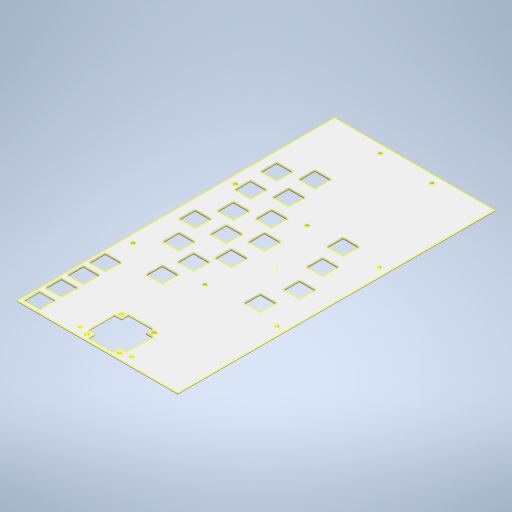
# Autodesk Inventor part: frame
Saved by Autodesk Inventor 2024 (Build 280153000, 153)
## iProperties
Created: 2023-10-17
Part Number: frame
Material: ABS 塑料
Document SubType Name: Modeling
Designer: Administrator
Density: 1.06 g/cm^3
Appearance: 白色
Author: Administrator
Autodesk Inventor part; units mm, degrees
(part 1 of 2)
ref_plane "YZ Plane" through (0, 0, 0) normal (1, 0, 0) x (0, 1, 0)
ref_plane "XY Plane" through (0, 0, 0) normal (0, 0, 1) x (1, 0, 0)
ref_plane "底层" through (0, -2, 0) normal (0, 1, 0) x (-1, 0, 0)
ref_plane "第二层" through (0, 4, 0) normal (0, 1, 0) x (-1, 0, 0)
ref_plane "第三层" through (0, 8, 0) normal (0, 1, 0) x (-1, 0, 0)
ref_plane "第四层" through (0, 12, 0) normal (0, 1, 0) x (-1, 0, 0)
sketch "第一层草图" plane through (0, 0, 0) normal (0, 1, 0) x (-1, 0, 0)
  line L0 (90, 150) -> (-90, 150)
  line L1 (-100, 140) -> (-100, -140)
  line L2 (-90, -150) -> (90, -150)
  line L3 (100, -140) -> (100, 140)
  line L4 (100, 150) -> (-100, -150) construction
  line L5 (-100, 150) -> (100, -150) construction
  arc A0 (100, 140) -> (90, 150) centre (90, 140) ccw
  arc A1 (-90, 150) -> (-100, 140) centre (-90, 140) ccw
  arc A2 (-100, -140) -> (-90, -150) centre (-90, -140) ccw
  arc A3 (90, -150) -> (100, -140) centre (90, -140) ccw
  point P0 (0, 0)
  dimension "d2" = 200
  dimension "d3" = 300
  dimension "d4" = 10
  constraints: 12 end point, 8 point on circle, 8 point on line, 8 tangent, 4 centre point, 3 equal radius, 2 midpoint, 2 parallel, 1 horizontal, 1 perpendicular
  measures "d2" distance of L5.end L4.end
  measures "d3" distance of L4.end L5.start
  measures "d4" radius of A0
sketch "第二层草图" plane through (0, 4, 0) normal (0, 1, 0) x (-1, 0, 0)
  line L0 (100, -140) -> (100, 140) projected
  line L1 (100, 0) -> (-88, 0)
  line L2 (90, 150) -> (-78, 150)
  line L3 (-88, 140) -> (-88, -140)
  line L4 (-78, -150) -> (90, -150)
  line L5 (100, -140) -> (100, 140)
  line L6 (100, 150) -> (-88, -150) construction
  line L7 (-88, 150) -> (100, -150) construction
  arc A0 (100, 140) -> (90, 150) centre (90, 140) ccw
  arc A1 (-78, 150) -> (-88, 140) centre (-78, 140) ccw
  arc A2 (-88, -140) -> (-78, -150) centre (-78, -140) ccw
  arc A3 (90, -150) -> (100, -140) centre (90, -140) ccw
  point P0 (0, 0)
  point P1 (6, 0)
  dimension "d101" = 188
  dimension "d102" = 188
  dimension "d103" = 300
  dimension "d104" = 10
  dimension "d125" = 10
  constraints: 14 end point, 8 point on circle, 8 point on line, 8 tangent, 4 centre point, 4 midpoint, 2 equal radius, 2 horizontal, 2 parallel, 1 perpendicular
  measures "d101" distance of L1.start L1.end
  measures "d102" distance of L7.end L6.end
  measures "d103" distance of L6.end L7.start
  measures "d104" radius of A0
  measures "d125" radius of A3
sketch "第三层草图" plane through (0, 8, 0) normal (0, 1, 0) x (-1, 0, 0)
  line L0 (100, -140) -> (100, 140) projected
  line L1 (100, 0) -> (-76, 0)
  line L2 (90, 150) -> (-66, 150)
  line L3 (-76, 140) -> (-76, -140)
  line L4 (-66, -150) -> (90, -150)
  line L5 (100, -140) -> (100, 140)
  line L6 (100, 150) -> (-76, -150) construction
  line L7 (-76, 150) -> (100, -150) construction
  arc A0 (100, 140) -> (90, 150) centre (90, 140) ccw
  arc A1 (-66, 150) -> (-76, 140) centre (-66, 140) ccw
  arc A2 (-76, -140) -> (-66, -150) centre (-66, -140) ccw
  arc A3 (90, -150) -> (100, -140) centre (90, -140) ccw
  point P0 (0, 0)
  point P1 (12, 0)
  dimension "d105" = 176
  dimension "d106" = 176
  dimension "d107" = 300
  dimension "d108" = 10
  constraints: 14 end point, 8 point on circle, 8 point on line, 8 tangent, 4 centre point, 4 midpoint, 3 equal radius, 2 horizontal, 2 parallel, 1 perpendicular
  measures "d105" distance of L1.start L1.end
  measures "d106" distance of L7.end L6.end
  measures "d107" distance of L6.end L7.start
  measures "d108" radius of A0
sketch "第四层草图" plane through (0, 12, 0) normal (0, 1, 0) x (-1, 0, 0)
  line L0 (100, -140) -> (100, 140) projected
  line L1 (100, 0) -> (-64, 0)
  line L2 (90, 150) -> (-54, 150)
  line L3 (-64, 140) -> (-64, -140)
  line L4 (-54, -150) -> (90, -150)
  line L5 (100, -140) -> (100, 140)
  line L6 (100, 150) -> (-64, -150) construction
  line L7 (-64, 150) -> (100, -150) construction
  arc A0 (100, 140) -> (90, 150) centre (90, 140) ccw
  arc A1 (-54, 150) -> (-64, 140) centre (-54, 140) ccw
  arc A2 (-64, -140) -> (-54, -150) centre (-54, -140) ccw
  arc A3 (90, -150) -> (100, -140) centre (90, -140) ccw
  point P0 (0, 0)
  point P1 (18, 0)
  dimension "d109" = 164
  dimension "d110" = 164
  dimension "d111" = 300
  dimension "d112" = 10
  dimension "d113" = 10
  constraints: 14 end point, 8 point on circle, 8 point on line, 8 tangent, 4 centre point, 4 midpoint, 2 equal radius, 2 horizontal, 2 parallel, 1 perpendicular
  measures "d109" distance of L1.start L1.end
  measures "d110" distance of L7.end L6.end
  measures "d111" distance of L6.end L7.start
  measures "d112" radius of A0
  measures "d113" radius of A2
sketch "底层草图" plane through (0, -2, 0) normal (0, 1, 0) x (-1, 0, 0)
  line L0 (98, 140) -> (98, -140)
  arc A0 (90, -148) -> (98, -140) centre (90, -140) ccw
  line L1 (90, -148) -> (-90, -148)
  arc A1 (-98, -140) -> (-90, -148) centre (-90, -140) ccw
  line L2 (-98, -140) -> (-98, 140)
  arc A2 (-90, 148) -> (-98, 140) centre (-90, 140) ccw
  line L3 (-90, 148) -> (90, 148)
  arc A3 (98, 140) -> (90, 148) centre (90, 140) ccw
  point P0 (0, 0)
  constraints: 8 end point, 8 point on circle, 4 centre point
extrude "拉伸25" add sketch "底层草图" along normal blind 2
extrude "拉伸26" add sketch "第一层草图" along normal blind 4 separate body
extrude "拉伸27" add sketch "第二层草图" along normal blind 4 separate body
extrude "拉伸28" add sketch "第三层草图" along normal blind 4 separate body
extrude "拉伸29" add sketch "第四层草图" along normal blind 4 separate body
sketch "草图20" plane through (0, 16, 0) normal (0, 1, 0) x (1, 0, 0)
  line L0 (-100, 140) -> (-100, -140) projected
  arc A0 (-100, -140) -> (-90, -150) centre (-90, -140) ccw projected
  line L1 (-90, -150) -> (54, -150) projected
  arc A1 (54, -150) -> (64, -140) centre (54, -140) ccw projected
  line L2 (64, -140) -> (64, 140) projected
  arc A2 (64, 140) -> (54, 150) centre (54, 140) ccw projected
  line L3 (54, 150) -> (-90, 150) projected
  arc A3 (-90, 150) -> (-100, 140) centre (-90, 140) ccw projected
  line L4 (-90, -140) -> (-92.1213, -142.1213)
  line L5 (-90, -140) -> (-87, -140) construction
  circle A4 centre (-92.1213, -142.1213) radius 2.75
  line L6 (-90, 140) -> (-92.1213, 142.1213)
  circle A5 centre (-92.1213, 142.1213) radius 2.75
  line L7 (54, -140) -> (56.1213, -142.1213)
  line L8 (54, -140) -> (57, -140) construction
  circle A6 centre (56.1213, -142.1213) radius 2.75
  line L9 (54, 140) -> (56.1213, 142.1213)
  circle A7 centre (56.1213, 142.1213) radius 2.75
  line L10 (-88, -138) -> (-88, 138)
  line L11 (-88, 138) -> (52, 138)
  line L12 (52, 138) -> (52, -138)
  line L13 (52, -138) -> (-88, -138)
  line L14 (-89.3713, -142.1213) -> (-90.7463, -144.5029)
  line L15 (-90.7463, -144.5029) -> (-93.4963, -144.5029)
  line L16 (-93.4963, -144.5029) -> (-94.8713, -142.1213)
  line L17 (-94.8713, -142.1213) -> (-93.4963, -139.7398)
  line L18 (-93.4963, -139.7398) -> (-90.7463, -139.7398)
  line L19 (-90.7463, -139.7398) -> (-89.3713, -142.1213)
  line L20 (-89.3713, 142.1213) -> (-90.7463, 139.7398)
  line L21 (-90.7463, 139.7398) -> (-93.4963, 139.7398)
  line L22 (-93.4963, 139.7398) -> (-94.8713, 142.1213)
  line L23 (-94.8713, 142.1213) -> (-93.4963, 144.5029)
  line L24 (-93.4963, 144.5029) -> (-90.7463, 144.5029)
  line L25 (-90.7463, 144.5029) -> (-89.3713, 142.1213)
  line L26 (58.8713, 142.1213) -> (57.4963, 139.7398)
  line L27 (57.4963, 139.7398) -> (54.7463, 139.7398)
  line L28 (54.7463, 139.7398) -> (53.3713, 142.1213)
  line L29 (53.3713, 142.1213) -> (54.7463, 144.5029)
  line L30 (54.7463, 144.5029) -> (57.4963, 144.5029)
  line L31 (57.4963, 144.5029) -> (58.8713, 142.1213)
  line L32 (58.8713, -142.1213) -> (57.4963, -144.5029)
  line L33 (57.4963, -144.5029) -> (54.7463, -144.5029)
  line L34 (54.7463, -144.5029) -> (53.3713, -142.1213)
  line L35 (53.3713, -142.1213) -> (54.7463, -139.7398)
  line L36 (54.7463, -139.7398) -> (57.4963, -139.7398)
  line L37 (57.4963, -139.7398) -> (58.8713, -142.1213)
  circle A8 centre (-92.1213, -142.1213) radius 1.6
  circle A9 centre (-92.1213, 142.1213) radius 1.6
  circle A10 centre (56.1213, -142.1213) radius 1.6
  circle A11 centre (56.1213, 142.1213) radius 1.6
  point P0 (0, 0)
  dimension "d128" = 5.5
  dimension "d130" = 5.5
  dimension "d132" = 5.5
  dimension "d134" = 5.5
  dimension "d126" = 3
  dimension "d127" = 135
  dimension "d129" = 3
  dimension "d131" = 45
  dimension "d133" = 3
  dimension "d135" = 12
  dimension "d136" = 3.2
  dimension "d137" = 3.2
  dimension "d138" = 3.2
  dimension "d139" = 3.2
  constraints: 68 end point, 12 coincident, 4 centre point, 4 horizontal alignment, 2 equal length, 2 horizontal, 63 other
  measures "d126" distance of L4.start L4.end
  measures "d127" angle of L4 L5
  measures "d129" distance of L6.start L6.end
  measures "d131" angle of L7 L8
  measures "d133" distance of L9.start L9.end
  measures "d135" distance between parallel lines of L0 L10
  measures "d136" diameter of A8
  measures "d137" diameter of A9
  measures "d138" diameter of A10
  measures "d139" diameter of A11
extrude "拉伸30" cut sketch "草图20" against normal up to surface (18 mm away) contours L10 L11 L12 L13 bodies 4 3 2
hole "四角固定孔" at (-92.1213, 16, 142.1213) at (-92.1213, 16, -142.1213) at (56.1213, 16, -142.1213) at (56.1213, 16, 142.1213) direction (0, -1, 0) diameter 3.2 end through all counterbore diameter 6.2 counterbore depth 1 bodies 5
extrude "六角通孔1" cut sketch "草图20" against normal through all contours L19 L14 L15 L16 L17 L18 | A8 bodies 4 3 2
extrude "六角通孔2" cut sketch "草图20" against normal through all contours L35 L36 L37 L32 L33 L34 | A10 bodies 4 3 2
extrude "六角通孔3" cut sketch "草图20" against normal through all contours L28 L29 L30 L31 L26 L27 | A11 bodies 4 3 2
extrude "六角通孔4" cut sketch "草图20" against normal through all contours L20 L21 L22 L23 L24 L25 | A9 bodies 4 3 2
sketch "第二层开孔草图" plane through (0, 8, 0) normal (0, 1, 0) x (1, 0, 0)
  line L0 (-100, 0) -> (-98, 0)
  line L1 (-100, 0) -> (-98, 0) construction
  line L2 (-98, 0) -> (-88, 0)
  line L3 (-98, -15) -> (-88, -15)
  line L4 (-88, -15) -> (-88, 15)
  line L5 (-88, 15) -> (-98, 15)
  line L6 (-98, 15) -> (-98, -15)
  line L7 (-98, -15) -> (-88, 15) construction
  line L8 (-88, -15) -> (-98, 15) construction
  line L9 (-100, -4.9) -> (-98, -4.9)
  line L10 (-98, -4.9) -> (-98, 4.9)
  line L11 (-98, 4.9) -> (-100, 4.9)
  line L12 (-100, 4.9) -> (-100, -4.9)
  line L13 (-100, -4.9) -> (-98, 4.9) construction
  line L14 (-98, -4.9) -> (-100, 4.9) construction
  line L15 (-88, 76.5) -> (-98, 76.5)
  line L16 (-98, 76.5) -> (-100, 76.5)
  line L17 (-98, 76.5) -> (-96, 76.5) construction
  line L18 (-98, 61.5) -> (-88, 61.5)
  line L19 (-88, 61.5) -> (-88, 91.5)
  line L20 (-88, 91.5) -> (-98, 91.5)
  line L21 (-98, 91.5) -> (-98, 61.5)
  line L22 (-98, 61.5) -> (-88, 91.5) construction
  line L23 (-88, 61.5) -> (-98, 91.5) construction
  line L24 (-100, 71.6) -> (-98, 71.6)
  line L25 (-98, 71.6) -> (-98, 81.4)
  line L26 (-98, 81.4) -> (-100, 81.4)
  line L27 (-100, 81.4) -> (-100, 71.6)
  line L28 (-100, 71.6) -> (-98, 81.4) construction
  line L29 (-98, 71.6) -> (-100, 81.4) construction
  line L30 (-88, 15) -> (-88, 61.5)
  line L31 (-88, 38.25) -> (-100, 38.25)
  line L32 (-100, 26.75) -> (-88, 26.75)
  line L33 (-88, 26.75) -> (-88, 49.75)
  line L34 (-88, 49.75) -> (-100, 49.75)
  line L35 (-100, 49.75) -> (-100, 26.75)
  line L36 (-100, 26.75) -> (-88, 49.75) construction
  line L37 (-88, 26.75) -> (-100, 49.75) construction
  line L38 (-91.2527, 26.75) -> (-92.6263, 24.3708)
  line L39 (-92.6263, 24.3708) -> (-95.3737, 24.3708)
  line L40 (-95.3737, 24.3708) -> (-96.7473, 26.75)
  line L41 (-96.7473, 26.75) -> (-95.3737, 29.1292)
  line L42 (-95.3737, 29.1292) -> (-92.6263, 29.1292)
  line L43 (-92.6263, 29.1292) -> (-91.2527, 26.75)
  line L44 (-91.2527, 49.75) -> (-92.6263, 47.3708)
  line L45 (-92.6263, 47.3708) -> (-95.3737, 47.3708)
  line L46 (-95.3737, 47.3708) -> (-96.7473, 49.75)
  line L47 (-96.7473, 49.75) -> (-95.3737, 52.1292)
  line L48 (-95.3737, 52.1292) -> (-92.6263, 52.1292)
  line L49 (-92.6263, 52.1292) -> (-91.2527, 49.75)
  line L50 (-88, -15) -> (-88, -26.75)
  line L51 (-88, -26.75) -> (-100, -26.75)
  line L52 (-88, 91.5) -> (-88, 103.25)
  line L53 (-88, 103.25) -> (-100, 103.25)
  line L54 (-91.2501, -26.75) -> (-92.625, -29.1315)
  line L55 (-92.625, -29.1315) -> (-95.375, -29.1315)
  line L56 (-95.375, -29.1315) -> (-96.7499, -26.75)
  line L57 (-96.7499, -26.75) -> (-95.375, -24.3685)
  line L58 (-95.375, -24.3685) -> (-92.625, -24.3685)
  line L59 (-92.625, -24.3685) -> (-91.2501, -26.75)
  line L60 (-91.2501, 103.25) -> (-92.625, 100.8685)
  line L61 (-92.625, 100.8685) -> (-95.375, 100.8685)
  line L62 (-95.375, 100.8685) -> (-96.7499, 103.25)
  line L63 (-96.7499, 103.25) -> (-95.375, 105.6315)
  line L64 (-95.375, 105.6315) -> (-92.625, 105.6315)
  line L65 (-92.625, 105.6315) -> (-91.2501, 103.25)
  point P0 (0, 0)
  point P1 (-93, 0)
  point P2 (-99, 0)
  point P3 (-93, 76.5)
  point P4 (-99, 76.5)
  point P5 (-94, 38.25)
  point P6 (-94, 26.75)
  point P7 (-94, 49.75)
  point P8 (-94, -26.75)
  point P9 (-94, 103.25)
  dimension "d164" = 2
  dimension "d165" = 0
  dimension "d166" = 30
  dimension "d167" = 9.8
  dimension "d172" = 10
  dimension "d173" = 2
  dimension "d174" = 180
  dimension "d175" = 10
  dimension "d176" = 30
  dimension "d177" = 2
  dimension "d178" = 9.8
  dimension "d183" = 23
  dimension "d189" = 11.75
  dimension "d190" = 11.75
  constraints: 132 end point, 10 midpoint, 2 collinear, 2 horizontal, 52 other
  measures "d164" distance of L0.start L0.end
  measures "d165" distance between parallel lines of L0 L1
  measures "d166" distance of L4.end L3.end
  measures "d167" distance of L10.end L9.end
  measures "d172" distance of L15.start L15.end
  measures "d173" distance of L16.start L16.end
  measures "d174" angle of L16 L17
  measures "d175" distance of L20.end L19.end
  measures "d176" distance of L19.end L18.end
  measures "d177" distance of L26.end L25.end
  measures "d178" distance of L25.end L24.end
  measures "d183" distance of L33.end L32.end
  measures "d189" distance of L50.start L50.end
  measures "d190" distance of L52.start L52.end
extrude "拉伸35" cut sketch "第二层开孔草图" against normal blind 10 contours L6 L5 L4 L2 | L2 L4 L3 L6 bodies 3 2
extrude "拉伸36" cut sketch "第二层开孔草图" against normal blind 10 contours L12 L11 L6 L0 | L0 L6 L9 L12 bodies 3
extrude "拉伸37" cut sketch "第二层开孔草图" against normal through all contours L19 L18 L21 L15 | L15 L21 L20 L19 bodies 3 2
extrude "拉伸38" cut sketch "第二层开孔草图" against normal through all contours L21 L24 L27 L16 | L16 L27 L26 L21 bodies 3
ref_plane "第三层开孔面" through (0, 12, 0) normal (0, 1, 0) x (1, 0, 0)
sketch "第三层开孔草图" plane through (0, 12, 0) normal (0, 1, 0) x (1, 0, 0)
  line L0 (-95.3737, 29.1292) -> (-92.6263, 29.1292) projected
  line L1 (-96.7473, 26.75) -> (-95.3737, 29.1292) projected
  line L2 (-95.3737, 24.3708) -> (-96.7473, 26.75) projected
  line L3 (-92.6263, 24.3708) -> (-95.3737, 24.3708) projected
  line L4 (-91.2527, 26.75) -> (-92.6263, 24.3708) projected
  line L5 (-92.6263, 29.1292) -> (-91.2527, 26.75) projected
  line L6 (-91.2527, 49.75) -> (-92.6263, 47.3708) projected
  line L7 (-92.6263, 47.3708) -> (-95.3737, 47.3708) projected
  line L8 (-95.3737, 47.3708) -> (-96.7473, 49.75) projected
  line L9 (-96.7473, 49.75) -> (-95.3737, 52.1292) projected
  line L10 (-95.3737, 52.1292) -> (-92.6263, 52.1292) projected
  line L11 (-92.6263, 52.1292) -> (-91.2527, 49.75) projected
  line L12 (-96.7499, -26.75) -> (-95.375, -24.3685) projected
  line L13 (-95.375, -29.1315) -> (-96.7499, -26.75) projected
  line L14 (-92.625, -29.1315) -> (-95.375, -29.1315) projected
  line L15 (-91.2501, -26.75) -> (-92.625, -29.1315) projected
  line L16 (-92.625, -24.3685) -> (-91.2501, -26.75) projected
  line L17 (-95.375, -24.3685) -> (-92.625, -24.3685) projected
  line L18 (-95.375, 100.8685) -> (-96.7499, 103.25) projected
  line L19 (-92.625, 100.8685) -> (-95.375, 100.8685) projected
  line L20 (-91.2501, 103.25) -> (-92.625, 100.8685) projected
  line L21 (-92.625, 105.6315) -> (-91.2501, 103.25) projected
  line L22 (-95.375, 105.6315) -> (-92.625, 105.6315) projected
  line L23 (-96.7499, 103.25) -> (-95.375, 105.6315) projected
  point P0 (0, 0)
extrude "中间层固定孔" cut sketch "第三层开孔草图" against normal through all bodies 4 3 2
sketch "底部孔草图" plane through (0, -2, 0) normal (0, -1, 0) x (1, 0, 0)
  circle A0 centre (-92.1213, -142.1213) radius 2.75 projected
  circle A1 centre (56.1213, -142.1213) radius 2.75 projected
  circle A2 centre (56.1213, 142.1213) radius 2.75 projected
  circle A3 centre (-92.1213, 142.1213) radius 2.75 projected
  line L0 (-96.7473, -26.75) -> (-95.3737, -24.3708) projected
  line L1 (-95.3737, -29.1292) -> (-96.7473, -26.75) projected
  line L2 (-92.6263, -29.1292) -> (-95.3737, -29.1292) projected
  line L3 (-91.2527, -26.75) -> (-92.6263, -29.1292) projected
  line L4 (-92.6263, -24.3708) -> (-91.2527, -26.75) projected
  line L5 (-95.3737, -24.3708) -> (-92.6263, -24.3708) projected
  line L6 (-95.375, 24.3685) -> (-96.7499, 26.75) projected
  line L7 (-96.7499, 26.75) -> (-95.375, 29.1315) projected
  line L8 (-95.375, 29.1315) -> (-92.625, 29.1315) projected
  line L9 (-92.625, 29.1315) -> (-91.2501, 26.75) projected
  line L10 (-91.2501, 26.75) -> (-92.625, 24.3685) projected
  line L11 (-92.625, 24.3685) -> (-95.375, 24.3685) projected
  circle A4 centre (-94, -26.75) radius 2.3792
  circle A5 centre (-94, 26.75) radius 2.3815
  point P0 (0, 0)
  constraints: 6 tangent, 2 centre point
hole "底板定位孔" at (-92.1213, -2, -142.1213) at (-92.1213, -2, 142.1213) at (56.1213, -2, 142.1213) at (56.1213, -2, -142.1213) at (-94, -2, -26.75) at (-94, -2, 26.75) direction (0, 1, 0) diameter 3.2 end through all counterbore diameter 6.6 counterbore depth 1 bodies 1
ref_plane "按键孔位平面" through (0, 16, 0) normal (0, 1, 0) x (1, 0, 0)
sketch "按键孔位图" plane through (0, 16, 0) normal (0, 1, 0) x (1, 0, 0)
  line L0 (-88, -138) -> (-88, -128)
  line L1 (-88, -128) -> (-78, -128)
  line L2 (-88, -128) -> (-78, -128) construction
  line L3 (-68.85, -137.15) -> (-68.85, -118.85)
  line L4 (-68.85, -118.85) -> (-87.15, -118.85)
  line L5 (-87.15, -118.85) -> (-87.15, -137.15)
  line L6 (-87.15, -137.15) -> (-68.85, -118.85) construction
  line L7 (-68.85, -137.15) -> (-87.15, -118.85) construction
  line L8 (-78, -128) -> (-78, -109)
  line L9 (-78, -109) -> (-78, -90)
  line L10 (-78, -90) -> (-78, -71)
  line L11 (-87.15, -118.15) -> (-68.85, -118.15)
  line L12 (-68.85, -118.15) -> (-68.85, -99.85)
  line L13 (-68.85, -99.85) -> (-87.15, -99.85)
  line L14 (-87.15, -99.85) -> (-87.15, -118.15)
  line L15 (-87.15, -118.15) -> (-68.85, -99.85) construction
  line L16 (-68.85, -118.15) -> (-87.15, -99.85) construction
  line L17 (-87.15, -99.15) -> (-68.85, -99.15)
  line L18 (-68.85, -99.15) -> (-68.85, -80.85)
  line L19 (-68.85, -80.85) -> (-87.15, -80.85)
  line L20 (-87.15, -80.85) -> (-87.15, -99.15)
  line L21 (-87.15, -99.15) -> (-68.85, -80.85) construction
  line L22 (-68.85, -99.15) -> (-87.15, -80.85) construction
  line L23 (-87.15, -80.15) -> (-68.85, -80.15)
  line L24 (-68.85, -80.15) -> (-68.85, -61.85)
  line L25 (-87.15, -61.85) -> (-87.15, -80.15)
  line L26 (-87.15, -80.15) -> (-68.85, -61.85) construction
  line L27 (-68.85, -80.15) -> (-87.15, -61.85) construction
  line L28 (-87.15, -137.15) -> (-68.85, -137.15)
  line L29 (-68.85, -61.85) -> (-87.15, -61.85)
  line L30 (-67.85, -60.85) -> (-67.85, -138.15)
  line L31 (-67.85, -138.15) -> (-88.15, -138.15)
  line L32 (-88.15, -138.15) -> (-88.15, -60.85)
  line L33 (-88.15, -60.85) -> (-67.85, -60.85)
  line L34 (-100, 140) -> (-100, -140) projected
  arc A0 (-100, -140) -> (-90, -150) centre (-90, -140) ccw projected
  line L35 (-90, -150) -> (54, -150) projected
  arc A1 (54, -150) -> (64, -140) centre (54, -140) ccw projected
  line L36 (64, -140) -> (64, 140) projected
  arc A2 (64, 140) -> (54, 150) centre (54, 140) ccw projected
  line L37 (54, 150) -> (-90, 150) projected
  arc A3 (-90, 150) -> (-100, 140) centre (-90, 140) ccw projected
  line L38 (-34.75, -135.5) -> (-1.25, -135.5)
  line L39 (-1.25, -135.5) -> (-1.25, -100.1)
  line L40 (-1.25, -100.1) -> (-34.75, -100.1)
  line L41 (-34.75, -100.1) -> (-34.75, -135.5)
  line L42 (-34.75, -117.8) -> (-28.4, -117.8)
  line L43 (-28.4, -117.8) -> (-11.7, -117.8)
  line L44 (-28.4, -133.51) -> (-11.7, -133.51)
  line L45 (-11.7, -133.51) -> (-11.7, -102.09)
  line L46 (-11.7, -102.09) -> (-28.4, -102.09)
  line L47 (-28.4, -102.09) -> (-28.4, -133.51)
  line L48 (-28.4, -133.51) -> (-11.7, -102.09) construction
  line L49 (-11.7, -133.51) -> (-28.4, -102.09) construction
  line L50 (-1.25, -135.5) -> (-3.75, -135.5)
  line L51 (-3.75, -135.5) -> (-3.75, -132.9)
  line L52 (-3.75, -132.9) -> (-1.25, -132.9)
  line L53 (-1.25, -132.9) -> (-1.25, -135.5)
  line L54 (-1.25, -100.1) -> (-3.75, -100.1)
  line L55 (-3.75, -100.1) -> (-3.75, -102.7)
  line L56 (-3.75, -102.7) -> (-1.25, -102.7)
  line L57 (-1.25, -102.7) -> (-1.25, -100.1)
  line L58 (-34.75, -135.5) -> (-32.25, -135.5)
  line L59 (-32.25, -135.5) -> (-32.25, -132.9)
  line L60 (-32.25, -132.9) -> (-34.75, -132.9)
  line L61 (-34.75, -132.9) -> (-34.75, -135.5)
  line L62 (-34.75, -100.1) -> (-32.25, -100.1)
  line L63 (-32.25, -100.1) -> (-32.25, -102.7)
  line L64 (-32.25, -102.7) -> (-34.75, -102.7)
  line L65 (-34.75, -102.7) -> (-34.75, -100.1)
  circle A4 centre (-32.25, -132.9) radius 1.5
  circle A5 centre (-32.25, -102.7) radius 1.5
  circle A6 centre (-3.75, -102.7) radius 1.5
  circle A7 centre (-3.75, -132.9) radius 1.5
  line L66 (-28.325, -129.3) -> (-34.825, -106.3) construction
  line L67 (-34.825, -129.3) -> (-28.325, -106.3) construction
  line L68 (-42.9444, -52.74) -> (-42.9444, -30.74) construction
  line L69 (-39.1242, -31.0742) -> (-39.1242, -9.0742) construction
  arc A8 (-26.335, -24.0516) -> (-36.8992, -16.6544) centre (-26.5055, -13.0529) ccw
  circle A9 centre (-24.3412, 13.6849) radius 11
  circle A10 centre (27.0645, -7.153) radius 13.5
  circle A11 centre (19.8671, -34.2122) radius 11
  circle A12 centre (19.8671, 19.9061) radius 11
  line L70 (19.8671, -34.2122) -> (27.0645, -7.153)
  line L71 (27.0645, -7.153) -> (19.8671, 19.9061)
  line L72 (-24.3412, 13.6849) -> (-0.0168, 13.6849) construction
  line L73 (-24.3412, 13.6849) -> (7.2272, 13.6849) construction
  line L74 (-24.3412, 13.6849) -> (7.2272, 13.6849) construction
  line L75 (-24.3412, 13.6849) -> (-38.6806, 34.1637)
  line L76 (-24.3412, 13.6849) -> (0.6588, 13.6849) construction
  line L77 (-38.6806, 34.1637) -> (-47.2311, 57.6561)
  line L78 (-47.2311, 57.6561) -> (-49.41, 82.5609)
  line L79 (-26.5055, -13.0529) -> (-39.9845, -32.3029)
  line L80 (-26.5055, -13.0529) -> (-3.0055, -13.0529) construction
  line L81 (-39.9845, -32.3029) -> (-44.0653, -55.4459)
  circle A13 centre (-38.6806, 34.1637) radius 11
  circle A14 centre (-47.2311, 57.6561) radius 11
  circle A15 centre (-49.41, 82.5609) radius 11
  circle A16 centre (-46.7695, 2.9431) radius 11
  line L82 (-46.7695, 2.9431) -> (-61.1089, 23.4219)
  line L83 (-61.1089, 23.4219) -> (-69.6594, 46.9142)
  line L84 (-69.6594, 46.9142) -> (-71.8383, 71.8191)
  circle A17 centre (-61.1089, 23.4219) radius 11
  circle A18 centre (-69.6594, 46.9142) radius 11
  circle A19 centre (-71.8383, 71.8191) radius 11
  circle A20 centre (-71.6744, 0.7642) radius 11
  line L85 (19.8671, 19.9061) -> (13.5007, 44.0819)
  circle A21 centre (13.5007, 44.0819) radius 11
  line L86 (-18, -138) -> (-34.75, -138)
  line L87 (-34.75, -138) -> (-34.75, -135.5)
  line L88 (-46.9494, -43.0088) -> (-46.9485, -43.0036)
  line L89 (-37.3423, -19.8122) -> (-37.3393, -19.8079)
  line L90 (-37.1013, -44.7453) -> (-37.1004, -44.7401)
  line L91 (-29.1508, -25.548) -> (-29.1477, -25.5436)
  arc A22 (-48.8681, -45.5498) -> (-36.1675, -47.7893) centre (-44.0653, -55.4459) ccw
  arc A23 (-35.1818, -42.1991) -> (-29.5908, -28.7014) centre (-39.9845, -32.3029) ccw
  arc A24 (-48.8681, -45.5498) -> (-46.9494, -43.0088) centre (-50.3962, -42.401) ccw
  arc A25 (-46.9485, -43.0036) -> (-47.8824, -39.9596) centre (-50.3953, -42.3958) ccw
  arc A26 (-37.1013, -44.7453) -> (-36.1675, -47.7893) centre (-33.6545, -45.3531) ccw
  arc A27 (-35.1818, -42.1991) -> (-37.1004, -44.7401) centre (-33.6536, -45.3478) ccw
  arc A28 (-40.1551, -21.3043) -> (-37.3423, -19.8122) centre (-40.2093, -17.8047) ccw
  arc A29 (-37.3393, -19.8079) -> (-36.8992, -16.6544) centre (-40.2063, -17.8003) ccw
  arc A30 (-29.1508, -25.548) -> (-29.5908, -28.7014) centre (-26.2838, -27.5555) ccw
  arc A31 (-26.335, -24.0516) -> (-29.1477, -25.5436) centre (-26.2807, -27.5511) ccw
  circle A32 centre (-92.1213, -142.1213) radius 1.6 projected
  circle A33 centre (-92.1213, 142.1213) radius 1.6 projected
  circle A34 centre (56.1213, -142.1213) radius 1.6 projected
  circle A35 centre (56.1213, 142.1213) radius 1.6 projected
  line L92 (-39.9845, -32.3029) -> (-61.6957, -23.3099)
  arc A36 (-50.9947, -20.7628) -> (-55.93, -32.6777) centre (-61.6957, -23.3099) ccw
  line L93 (-42.9221, -36.4982) -> (-42.9444, -36.4889)
  line L94 (-52.7511, -32.4268) -> (-52.756, -32.4248)
  line L95 (-39.0952, -27.2594) -> (-39.1242, -27.2474)
  line L96 (-48.9243, -23.188) -> (-48.9292, -23.186)
  arc A37 (-40.1551, -21.3043) -> (-45.7503, -22.9351) centre (-39.9845, -32.3029) ccw
  arc A38 (-50.6856, -34.85) -> (-47.8824, -39.9596) centre (-39.9845, -32.3029) ccw
  arc A39 (-50.9947, -20.7628) -> (-48.9292, -23.186) centre (-47.5898, -19.9524) ccw
  arc A40 (-48.9243, -23.188) -> (-45.7503, -22.9351) centre (-47.5849, -19.9545) ccw
  arc A41 (-52.756, -32.4248) -> (-55.93, -32.6777) centre (-54.0954, -35.6584) ccw
  arc A42 (-50.6856, -34.85) -> (-52.7511, -32.4268) centre (-54.0905, -35.6604) ccw
  line L97 (-34.75, -135.5) -> (-28.75, -135.5)
  line L98 (-28.75, -135.5) -> (-28.75, -129.5)
  line L99 (-28.75, -129.5) -> (-34.75, -129.5)
  line L100 (-34.75, -129.5) -> (-34.75, -135.5)
  line L101 (-34.75, -100.1) -> (-28.75, -100.1)
  line L102 (-28.75, -100.1) -> (-28.75, -106.1)
  line L103 (-28.75, -106.1) -> (-34.75, -106.1)
  line L104 (-34.75, -106.1) -> (-34.75, -100.1)
  line L105 (-1.25, -135.5) -> (-7.25, -135.5)
  line L106 (-7.25, -135.5) -> (-7.25, -129.5)
  line L107 (-7.25, -129.5) -> (-1.25, -129.5)
  line L108 (-1.25, -129.5) -> (-1.25, -135.5)
  line L109 (-1.25, -100.1) -> (-7.25, -100.1)
  line L110 (-7.25, -100.1) -> (-7.25, -106.1)
  line L111 (-7.25, -106.1) -> (-1.25, -106.1)
  line L112 (-1.25, -106.1) -> (-1.25, -100.1)
  point P0 (-20.05, -117.8)
  point P1 (-31.575, -117.8)
  point P2 (-47.2879, -44.9286)
  point P3 (-38.4604, -21.409)
  point P4 (-37.4398, -46.6651)
  point P5 (-28.0296, -23.9468)
  point P6 (-46.61, -41.0838)
  point P7 (-36.7619, -42.8203)
  point P8 (-30.2689, -27.1448)
  point P9 (-36.2211, -18.211)
  point P10 (-50.7302, -22.44)
  point P11 (-50.9501, -33.1728)
  point P12 (-54.557, -31.6788)
  point P13 (-47.1233, -23.934)
  dimension "d195" = 10
  dimension "d196" = 10
  dimension "d197" = 0
  dimension "d198" = 18.3
  dimension "d199" = 18.3
  dimension "d200" = 19
  dimension "d202" = 19
  dimension "d203" = 19
  dimension "d204" = 18.3
  dimension "d205" = 18.3
  dimension "d206" = 18.3
  dimension "d207" = 18.3
  dimension "d208" = 18.3
  dimension "d209" = 18.3
  dimension "d288" = 33.5
  dimension "d289" = 35.4
  dimension "d290" = 6.35
  dimension "d291" = 16.7
  dimension "d292" = 16.7
  dimension "d293" = 31.42
  dimension "d294" = 2.5
  dimension "d295" = 2.6
  dimension "d296" = 2.5
  dimension "d297" = 2.6
  dimension "d298" = 2.5
  dimension "d299" = 2.6
  dimension "d300" = 2.5
  dimension "d301" = 2.6
  dimension "d302" = 3
  dimension "d303" = 3
  dimension "d304" = 3
  dimension "d305" = 3
  dimension "d307" = 23
  dimension "d363" = 22
  dimension "d364" = 22
  dimension "d365" = 27
  dimension "d366" = 22
  dimension "d367" = 22
  dimension "d381" = 25
  dimension "d382" = 125
  dimension "d383" = 25
  dimension "d384" = 165
  dimension "d385" = 25
  dimension "d386" = 165
  dimension "d387" = 23.5
  dimension "d388" = 125
  dimension "d389" = 23.5
  dimension "d390" = 155
  dimension "d393" = 22
  dimension "d394" = 22
  dimension "d395" = 22
  dimension "d408" = 22
  dimension "d409" = 25
  dimension "d410" = 25
  dimension "d411" = 165
  dimension "d412" = 25
  dimension "d413" = 165
  dimension "d414" = 22
  dimension "d415" = 22
  dimension "d416" = 22
  dimension "d420" = 22
  dimension "d423" = 25
  dimension "d424" = 22
  dimension "d425" = 16.75
  constraints: 218 end point, 46 point on circle, 35 centre point, 22 tangent, 17 point on line, 12 midpoint, 8 coincident, 7 equal radius, 6 horizontal, 4 parallel, 3 equal length
  measures "d195" distance of L0.start L0.end
  measures "d196" distance of L1.start L1.end
  measures "d197" distance between parallel lines of L1 L2
  measures "d198" distance of L4.end L3.end
  measures "d199" distance of L3.end L3.start
  measures "d200" distance of L8.start L8.end
  measures "d202" distance of L9.start L9.end
  measures "d203" distance of L10.start L10.end
  measures "d204" distance of L13.end L12.end
  measures "d205" distance of L12.end L11.end
  measures "d206" distance of L19.end L18.end
  measures "d207" distance of L18.end L17.end
  measures "d208" distance of L25.start L24.end
  measures "d209" distance of L24.end L23.end
  measures "d288" distance of L40.end L39.end
  measures "d289" distance of L39.end L38.end
  measures "d290" distance of L42.start L42.end
  measures "d291" distance of L43.start L43.end
  measures "d292" distance of L46.end L45.end
  measures "d293" distance of L45.end L44.end
  measures "d294" distance of L51.end L52.end
  measures "d295" distance of L50.end L51.end
  measures "d296" distance of L56.end L55.end
  measures "d297" distance of L55.end L54.end
  measures "d298" distance of L60.end L59.end
  measures "d299" distance of L59.end L58.end
  measures "d300" distance of L63.end L64.end
  measures "d301" distance of L62.end L63.end
  measures "d302" diameter of A4
  measures "d303" diameter of A5
  measures "d304" diameter of A6
  measures "d305" diameter of A7
  measures "d307" distance of L67.start L66.end
  measures "d363" diameter of A8
  measures "d364" diameter of A9
  measures "d365" diameter of A10
  measures "d366" diameter of A11
  measures "d367" diameter of A12
  measures "d381" distance of L72.start L75.end
  measures "d382" angle of L76 L75
  measures "d383" distance of L75.end L77.end
  measures "d384" angle of L75 L77
  measures "d385" distance of L77.end L78.end
  measures "d386" angle of L77 L78
  measures "d387" distance of L79.start L79.end
  measures "d388" angle of L79 L80
  measures "d389" distance of L79.end L81.end
  measures "d390" angle of L81 L79
  measures "d393" diameter of A13
  measures "d394" diameter of A14
  measures "d395" diameter of A15
  measures "d408" diameter of A16
  measures "d409" distance of L82.start L83.start
  measures "d410" distance of L83.start L84.start
  measures "d411" angle of L82 L83
  measures "d412" distance of L84.start L84.end
  measures "d413" angle of L83 L84
  measures "d414" diameter of A17
  measures "d415" diameter of A18
  measures "d416" diameter of A19
  measures "d420" diameter of A20
  measures "d423" distance of L71.end L85.end
  measures "d424" diameter of A21
  measures "d425" distance of L86.start L86.end
extrude "按键开孔" cut sketch "按键孔位图" against normal through all contours L5 L4 L8 L1 | L1 L8 L4 L3 L28 L5 | L11 L14 L13 L9 L8 | L8 L9 L13 L12 L11 | L17 L20 L19 L10 L9 | L9 L10 L19 L18 L17 | L25 L29 L24 L23 | L30 L31 L32 L33 | A31 L91 A30 A23 A27 L90 A26 A22 A24 L88 A25 A38 A42 L94 A41 A36 A39 L96 A40 A37 A28 L89 A29 A8 | A9 | A10 L70 L71 | L71 L70 A10 | A11 | A12 L71 L85 | L85 L71 A12 | A13 L77 L75 | L75 L77 A13 | A14 L78 L77 | L77 L78 A14 | A15 | A16 | A17 L83 L82 | L82 L83 A17 | A18 L84 L83 | L83 L84 A18 | A19 | A20 bodies 5
ref_plane "PCB平面" through (0, 3.5, 0) normal (0, 1, 0) x (1, 0, 0)
sketch "PCB轮廓草图" plane through (0, 3.5, 0) normal (0, 1, 0) x (1, 0, 0)
  line L0 (-88, -138) -> (-88, -15) projected
  line L1 (-88, -15) -> (-98, -15) projected
  line L2 (-98, -15) -> (-98, 15) projected
  line L3 (-98, 15) -> (-88, 15) projected
  line L4 (-88, 15) -> (-88, 61.5) projected
  line L5 (-88, 61.5) -> (-98, 61.5) projected
  line L6 (-98, 61.5) -> (-98, 91.5) projected
  line L7 (-98, 91.5) -> (-88, 91.5) projected
  line L8 (-88, 91.5) -> (-88, 138) projected
  line L9 (-88, 138) -> (52, 138) projected
  line L10 (52, 138) -> (52, -138) projected
  line L11 (52, -138) -> (-88, -138) projected
  line L12 (-87.5, -14.5) -> (-87.5, -137.5)
  line L13 (-87.5, -137.5) -> (51.5, -137.5)
  line L14 (51.5, -137.5) -> (51.5, 137.5)
  line L15 (51.5, 137.5) -> (-87.5, 137.5)
  line L16 (-87.5, 137.5) -> (-87.5, 91)
  line L17 (-87.5, 91) -> (-97.5, 91)
  line L18 (-97.5, 91) -> (-97.5, 62)
  line L19 (-97.5, 62) -> (-87.5, 62)
  line L20 (-87.5, 62) -> (-87.5, 14.5)
  line L21 (-87.5, 14.5) -> (-97.5, 14.5)
  line L22 (-97.5, 14.5) -> (-97.5, -14.5)
  line L23 (-97.5, -14.5) -> (-87.5, -14.5)
  line L24 (-87.5, -137.5) -> (-80.4289, -130.4289)
  line L25 (-87.5, -137.5) -> (-77.5, -137.5) construction
  line L26 (51.5, -137.5) -> (44.4289, -130.4289)
  line L27 (51.5, -137.5) -> (61.5, -137.5) construction
  line L28 (51.5, 137.5) -> (44.4289, 130.4289)
  line L29 (51.5, 137.5) -> (61.5, 137.5) construction
  line L30 (-87.5, 137.5) -> (-80.4289, 130.4289)
  line L31 (-87.5, 137.5) -> (-77.5, 137.5) construction
  line L32 (-80.4289, -130.4289) -> (-40.4289, -130.4289)
  line L33 (-80.4289, -130.4289) -> (-40.4289, -130.4289) construction
  line L34 (44.4289, -130.4289) -> (4.4289, -130.4289)
  line L35 (44.4289, -130.4289) -> (84.4289, -130.4289) construction
  line L36 (-80.4289, 130.4289) -> (-40.4289, 130.4289)
  line L37 (-80.4289, 130.4289) -> (-40.4289, 130.4289) construction
  line L38 (44.4289, 130.4289) -> (4.4289, 130.4289)
  line L39 (44.4289, -130.4289) -> (44.4289, -44.4289)
  line L40 (44.4289, -130.4289) -> (130.4289, -130.4289) construction
  line L41 (44.4289, 130.4289) -> (44.4289, 44.4289)
  line L42 (44.4289, 130.4289) -> (130.4289, 130.4289) construction
  line L43 (-97.5, -14.5) -> (-93.9645, -10.9645)
  line L44 (-97.5, 14.5) -> (-93.9645, 10.9645)
  line L45 (-97.5, 62) -> (-93.9645, 65.5355)
  line L46 (-97.5, 91) -> (-93.9645, 87.4645)
  line L47 (-80.4289, -130.4289) -> (-80.4289, -44.4289)
  circle A0 centre (-80.4289, -44.4289) radius 1.5
  circle A1 centre (-40.4289, -130.4289) radius 1.5
  circle A2 centre (4.4289, -130.4289) radius 1.5
  circle A3 centre (44.4289, -44.4289) radius 1.5
  circle A4 centre (44.4289, 44.4289) radius 1.5
  circle A5 centre (4.4289, 130.4289) radius 1.5
  circle A6 centre (-40.4289, 130.4289) radius 1.5
  circle A7 centre (-93.9645, -10.9645) radius 1.5
  circle A8 centre (-93.9645, 10.9645) radius 1.5
  circle A9 centre (-93.9645, 65.5355) radius 1.5
  circle A10 centre (-93.9645, 87.4645) radius 1.5
  line L48 (44.4289, -44.4289) -> (-18.0001, -44.4289)
  line L49 (44.4289, 44.4289) -> (-18.0001, 44.4289)
  circle A11 centre (-18.0001, -44.4289) radius 1.5
  circle A12 centre (-18.0001, 44.4289) radius 1.5
  line L50 (-80.4289, 130.4289) -> (-80.4289, 44.4289)
  circle A13 centre (-80.4289, 44.4289) radius 1.5
  point P0 (0, 0)
  dimension "d214" = 0.5
  dimension "d215" = 10
  dimension "d216" = 45
  dimension "d217" = 10
  dimension "d218" = 135
  dimension "d219" = 10
  dimension "d220" = 135
  dimension "d221" = 10
  dimension "d222" = 45
  dimension "d223" = 40
  dimension "d225" = 40
  dimension "d227" = 40
  dimension "d228" = 0
  dimension "d229" = 40
  dimension "d230" = 86
  dimension "d231" = 90
  dimension "d232" = 86
  dimension "d233" = 90
  dimension "d234" = 5
  dimension "d235" = 5
  dimension "d236" = 5
  dimension "d237" = 5
  dimension "d238" = 86
  dimension "d239" = 3
  dimension "d240" = 3
  dimension "d241" = 3
  dimension "d242" = 3
  dimension "d243" = 3
  dimension "d244" = 3
  dimension "d245" = 3
  dimension "d246" = 3
  dimension "d247" = 3
  dimension "d248" = 3
  dimension "d249" = 3
  dimension "d250" = 62.429
  dimension "d251" = 62.429
  dimension "d252" = 3
  dimension "d253" = 3
  dimension "d257" = 86
  dimension "d258" = 3
  constraints: 78 end point, 14 centre point, 9 equal length, 9 horizontal, 11 other
  measures "d214" distance between parallel lines of L0 L12
  measures "d215" distance of L24.start L24.end
  measures "d216" angle of L25 L24
  measures "d217" distance of L26.start L26.end
  measures "d218" angle of L27 L26
  measures "d219" distance of L28.start L28.end
  measures "d220" angle of L28 L29
  measures "d221" distance of L30.start L30.end
  measures "d222" angle of L30 L31
  measures "d223" distance of L32.start L32.end
  measures "d225" distance of L34.start L34.end
  measures "d227" distance of L36.start L36.end
  measures "d228" distance between parallel lines of L36 L37
  measures "d229" distance of L38.start L38.end
  measures "d230" distance of L39.start L39.end
  measures "d231" angle of L40 L39
  measures "d232" distance of L41.start L41.end
  measures "d233" angle of L41 L42
  measures "d234" distance of L43.start L43.end
  measures "d235" distance of L44.start L44.end
  measures "d236" distance of L45.start L45.end
  measures "d237" distance of L46.start L46.end
  measures "d238" distance of L47.start L47.end
  measures "d239" diameter of A0
  measures "d240" diameter of A1
  measures "d241" diameter of A2
  measures "d242" diameter of A3
  measures "d243" diameter of A4
  measures "d244" diameter of A5
  measures "d245" diameter of A6
  measures "d246" diameter of A7
  measures "d247" diameter of A8
  measures "d248" diameter of A9
  measures "d249" diameter of A10
  measures "d250" distance of L48.start L48.end
  measures "d251" distance of L49.start L49.end
  measures "d252" diameter of A11
  measures "d253" diameter of A12
  measures "d257" distance of L50.start L50.end
  measures "d258" diameter of A13
extrude "拉伸41" add sketch "PCB轮廓草图" against normal blind 1.2 separate body contours L23 L22 L21 L20 L19 L18 L17 L16 L15 L14 L13 L12 | A3 L48 L39 | L39 L48 A3 | A4 L49 L41 | L41 L49 A4 | A0 | A1 | A2 | A5 | A6 | A7 | A8 | A9 | A10 | A11 | A12 | A13
ref_plane "pisition平面" through (0, 8.5, 0) normal (0, 1, 0) x (1, 0, 0)